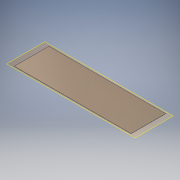
# Autodesk Inventor part: Base Gabinete
Saved by Autodesk Inventor 2017 (Build 210142000, 142)
## iProperties
Created: 2019-06-18
Part Number: Base Gabinete
Material: Stainless Steel
Document SubType Name: Sheet Metal
Designer: leonardo.prado
Density: 8 g/cm^3
Sheet Metal Rule: Default_mm
Appearance: Semi-Polished
Author: leonardo.prado
Autodesk Inventor part; units mm, degrees
ref_plane "YZ Plane" through (0, 0, 0) normal (1, 0, 0) x (0, 1, 0)
ref_plane "XZ Plane" through (0, 0, 0) normal (0, 1, 0) x (-1, 0, 0)
ref_plane "XY Plane" through (0, 0, 0) normal (0, 0, 1) x (1, 0, 0)
ref_plane "Work Plane1" through (0, 0, 0) normal (0, 0, 1) x (1, 0, 0)
sketch "Sketch1" plane through (0, 0, 0) normal (0, 0, 1) x (1, 0, 0)
  line L0 (468.299, 130) -> (468.299, 128.5)
  line L1 (-468.299, -145.7383) -> (-468.299, 128.5)
  line L2 (465.7383, -148.299) -> (-465.7383, -148.299)
  line L3 (-468.299, -148.299) -> (468.299, -148.299)
  line L4 (468.299, -148.299) -> (468.299, 130)
  line L5 (468.299, 130) -> (-468.299, 130)
  line L6 (-468.299, 130) -> (-468.299, -148.299)
  point P0 (0, 0)
extrude "Plate1" add sketch "Sketch1" against normal blind 1.5
equation "\"BendRadius\" = Thickness"
equation "\"BendReliefWidth\" = Thickness"
equation "\"BendReliefDepth\" = 0.5 * Thickness"
equation "\"CornerReliefSize\" = 4 * Thickness"
equation "\"MinimumRemnant\" = 2 * Thickness"
equation "\"TransitionRadius\" = BendRadius"
equation "\"JacobiRadiusSize\" = BendRadius"
equation "\"GapSize\" = Thickness"
equation "\"d0\" = BendRadius"
equation "\"Thickness\" = 1.5"
body "Solid1"
